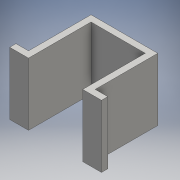
# Autodesk Inventor part: imu_case_2
Saved by Autodesk Inventor 2016 (Build 200138000, 138)
## iProperties
Created: 2015-11-15
Part Number: imu_case_2
Material: Generic
Document SubType Name: Modeling
Designer: Qiuyang
Density: 1 g/cm^3
Appearance: Default
Author: Qiuyang
Autodesk Inventor part; units mm, degrees
ref_plane "YZ Plane" through (0, 0, 0) normal (1, 0, 0) x (0, 1, 0)
ref_plane "XZ Plane" through (0, 0, 0) normal (0, 1, 0) x (-1, 0, 0)
ref_plane "XY Plane" through (0, 0, 0) normal (0, 0, 1) x (1, 0, 0)
sketch "Sketch2" plane through (0, 0, 0) normal (0, 0, 1) x (1, 0, 0)
  line L0 (0, 0) -> (6, 0)
  line L1 (6, 0) -> (6, 3)
  line L2 (6, 3) -> (0, 3)
  line L3 (0, 3) -> (0, 0)
  line L4 (6, 0) -> (9, 0)
  line L5 (9, 0) -> (9, 30)
  line L6 (9, 30) -> (6, 30)
  line L7 (6, 30) -> (6, 0)
  line L8 (6, 30) -> (38, 30)
  line L9 (38, 30) -> (38, 33)
  line L10 (38, 33) -> (6, 33)
  line L11 (6, 33) -> (6, 30)
  line L12 (38, 30) -> (35, 30)
  line L13 (35, 30) -> (35, 0)
  line L14 (35, 0) -> (38, 0)
  line L15 (38, 0) -> (38, 30)
  line L16 (38, 0) -> (44, 0)
  line L17 (44, 0) -> (44, 3)
  line L18 (44, 3) -> (38, 3)
  line L19 (38, 3) -> (38, 0)
  dimension "d0" = 6
  dimension "d1" = 3
  dimension "d2" = 3
  dimension "d3" = 30
  dimension "d4" = 32
  dimension "d5" = 3
  dimension "d6" = 3
  dimension "d7" = 30
  dimension "d8" = 6
  dimension "d9" = 3
  constraints: 40 end point, 10 parallel, 5 horizontal, 5 perpendicular
  measures "d0" distance of L2.end L1.end
  measures "d1" distance of L1.end L0.end
  measures "d2" distance of L6.end L5.end
  measures "d3" distance of L5.end L4.end
  measures "d4" distance of L10.end L9.end
  measures "d5" distance of L9.end L8.end
  measures "d6" distance of L14.end L13.end
  measures "d7" distance of L13.end L12.end
  measures "d8" distance of L18.end L17.end
  measures "d9" distance of L17.end L16.end
extrude "Extrusion1" add sketch "Sketch2" along normal blind 30
body "Solid1"
